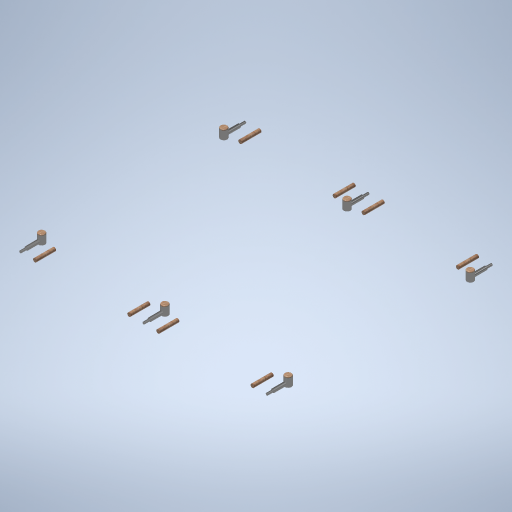
# Autodesk Inventor part: REC_01
Saved by Autodesk Inventor 2024.3 (Build 283343000, 343)
## iProperties
RuleStatus: InUse
Created: 2014-05-08
Part Number: REC_01
Material: Generic
Document SubType Name: Modeling
Designer: SauliusD
Density: 1 g/cm^3
Appearance: Default
Description: Pillar Board & 2 Nestled Boards from Sides Minifixes-01
AfterDocNew0: Fire Form
Author: SauliusD
Autodesk Inventor part; units mm, degrees
sketch "Sketch2" plane through (0, 0, 0) normal (0, 0, 1) x (1, 0, 0)
  line L0 (687.7589, -308.1253) -> (141.7589, -308.1253)
  line L1 (141.7589, -308.1253) -> (141.7589, 161.8747)
  line L2 (141.7589, 161.8747) -> (687.7589, 161.8747)
  line L3 (687.7589, 161.8747) -> (687.7589, -308.1253)
  point P0 (414.7589, 161.8747)
  point P1 (141.7589, -73.1253)
  constraints: 8 end point, 2 midpoint, 2 parallel, 1 horizontal, 1 perpendicular
ref_plane "Work Plane1" through (0, 0, -12.5) normal (0, 0, 1) x (1, 0, 0)
sketch "Sketch3" plane through (0, 0, -12.5) normal (0, 0, 1) x (1, 0, 0)
  line L0 (687.7589, 161.8747) -> (687.7589, -308.1253) construction
  line L1 (141.7589, 161.8747) -> (687.7589, 161.8747) construction
  line L2 (141.7589, -308.1253) -> (141.7589, 161.8747) construction
  line L3 (142.7589, 161.8747) -> (146.7589, 161.8747)
  line L4 (146.7589, 161.8747) -> (146.7589, 127.8747)
  line L5 (146.7589, 127.8747) -> (142.7589, 127.8747)
  line L6 (142.7589, 127.8747) -> (142.7589, 161.8747)
  line L7 (142.7589, 161.8747) -> (145.2589, 161.8747)
  line L8 (145.2589, 161.8747) -> (145.2589, 174.8747)
  line L9 (145.2589, 174.8747) -> (142.7589, 174.8747)
  line L10 (142.7589, 174.8747) -> (142.7589, 161.8747)
  line L11 (414.7589, 161.8747) -> (414.7589, 132.7708) construction
  line L12 (686.7589, 127.8747) -> (686.7589, 161.8747)
  point P0 (0, 0)
  dimension "d5" = 8
  dimension "d7" = 5
  dimension "d8" = 13
  dimension "Dist_Between_Planes" = 546
  dimension "Distance_between_Axis" = 544
  constraints: 20 end point, 5 parallel, 2 horizontal, 2 perpendicular, 2 symmetric about line, 1 collinear, 1 midpoint, 1 vertical alignment
  measures "d5" diameter of L4 L6
  measures "d7" diameter of L8 L10
  measures "d8" distance of L7.end L8.end
  measures "Dist_Between_Planes" distance of L1.start L0.start
  measures "Distance_between_Axis" distance between parallel lines of L6 L12
revolve "Minifix Revolve" add sketch "Sketch3" angle 360 about axis through (142.7589, 174.8747, -12.5) along (0, -1, 0)
sketch "Sketch4" plane through (0, 0, -12.5) normal (0, 0, 1) x (1, 0, 0)
  line L0 (138.7589, 127.8747) -> (146.7589, 127.8747) construction
  circle A0 centre (142.7589, 127.8747) radius 7.5
  point P0 (0, 0)
  dimension "d10" = 15
  constraints: 1 centre point, 1 midpoint
  measures "d10" diameter of A0
extrude "Minifix Extrude" add sketch "Sketch4" along normal up to surface (12.5 mm away)
extrude "Minifix extrude 2" add sketch "Sketch4" against normal blind 6
ref_plane "Work Plane2" through (414.7589, 161.8747, 0) normal (1, 0, 0) x (0, 1, 0)
ref_plane "Work Plane3" through (141.7589, -73.1253, 0) normal (0, 1, 0) x (-1, 0, 0)
sketch "Sketch5" plane through (0, 0, -12.5) normal (0, 0, 1) x (1, 0, 0)
  line L0 (142.7589, 271.4747) -> (142.7589, -404.7253) construction
  line L1 (174.7589, 174.8747) -> (174.7589, 131.8747)
  line L2 (174.7589, 174.8747) -> (178.7589, 174.8747)
  line L3 (178.7589, 174.8747) -> (178.7589, 131.8747)
  line L4 (178.7589, 131.8747) -> (174.7589, 131.8747)
  line L5 (140.2589, 174.8747) -> (145.2589, 174.8747) construction
  line L6 (138.7589, 161.8747) -> (146.7589, 161.8747) construction
  point P0 (0, 0)
  dimension "Dowel_D" = 8
  dimension "Dowel_Drill_Depth" = 30
  dimension "d17" = 32
  constraints: 8 end point, 2 parallel, 2 perpendicular, 1 collinear
  measures "Dowel_D" diameter of L3 L1
  measures "Dowel_Drill_Depth" distance between parallel lines of L4 L6
  measures "d17" distance from line of L1.start L0
revolve "Dowel Revolve" add sketch "Sketch5" angle 360 about axis through (174.7589, 174.8747, -12.5) along (0, -1, 0) separate body
mirror "Mirror1" about plane through (414.7589, 161.8747, 0) normal (1, 0, 0) of "Minifix Extrude", "Minifix Revolve", "Dowel Revolve", "Minifix extrude 2" bodies 1
sketch "Sketch6" plane through (0, 0, -12.5) normal (0, 0, 1) x (1, 0, 0)
  point P0 (0, 0)
sketch "Sketch7" plane through (0, 0, -12.5) normal (0, 0, 1) x (1, 0, 0)
  line L0 (414.7589, 271.4747) -> (414.7589, -404.7253) construction
  line L1 (417.2589, 161.8747) -> (414.7589, 161.8747)
  line L2 (414.7589, 161.8747) -> (414.7589, 174.8747)
  line L3 (414.7589, 174.8747) -> (417.2589, 174.8747)
  line L4 (417.2589, 174.8747) -> (417.2589, 161.8747)
  line L5 (414.7589, 161.8747) -> (418.7589, 161.8747)
  line L6 (418.7589, 161.8747) -> (418.7589, 127.8747)
  line L7 (418.7589, 127.8747) -> (414.7589, 127.8747)
  line L8 (414.7589, 127.8747) -> (414.7589, 161.8747)
  line L9 (140.2589, 174.8747) -> (145.2589, 174.8747) construction
  line L10 (138.7589, 161.8747) -> (146.7589, 161.8747) construction
  point P0 (0, 0)
  point P1 (414.7589, -404.7253)
  dimension "d19" = 34
  dimension "d20" = 5
  dimension "d21" = 8
  constraints: 16 end point, 4 parallel, 2 collinear, 2 horizontal, 2 perpendicular, 1 vertical, 1 other
  measures "d19" distance of L5.end L6.end
  measures "d20" diameter of L4 L2
  measures "d21" diameter of L6 L2
revolve "Center minixix Revolution" add sketch "Sketch7" angle 360 about axis through (414.7589, 161.8747, -12.5) along (0, 1, 0) separate body
sketch "Sketch8" plane through (0, 0, -12.5) normal (0, 0, 1) x (1, 0, 0)
  circle A0 centre (414.7589, 127.8747) radius 7.5
  line L0 (418.7589, 127.8747) -> (414.7589, 127.8747) construction
  point P0 (0, 0)
  dimension "d23" = 15
  constraints: 1 centre point, 1 coincident
  measures "d23" diameter of A0
extrude "Center minixix Extrusion 1" add sketch "Sketch8" along normal up to surface (12.5 mm away) bodies 3
extrude "Center minixix Extrusion 2" add sketch "Sketch8" against normal up to surface (6 mm away) bodies 3
ref_plane "Work Plane4" through (687.7589, 161.8747, 0) normal (0, 1, 0) x (-1, 0, 0)
mirror "Mirror2" about plane through (141.7589, -73.1253, 0) normal (0, 1, 0) of "Minifix Extrude", "Minifix Revolve", "Dowel Revolve", "Minifix extrude 2", "Mirror1" bodies 1
mirror "Mirror Center" about plane through (141.7589, -73.1253, 0) normal (0, 1, 0) of "Center minixix Revolution", "Center minixix Extrusion 1", "Center minixix Extrusion 2" bodies 3
sketch "Sketch9" plane through (142.7589, 127.8747, 0) normal (0, 0, 1) x (1, 0, 0)
  circle A0 centre (0, 0) radius 7.5 projected
  point P0 (-142.7589, -127.8747)
extrude "Side Cover Cap Extrusion" add sketch "Sketch9" along normal blind 2 separate body
fillet "Side Cover Cap Fillet" radius 1.6 1 edges at (135.2589, 127.8747, 2)
mirror "Mirror3" about plane through (414.7589, 161.8747, 0) normal (1, 0, 0) of "Side Cover Cap Extrusion", "Side Cover Cap Fillet" bodies 4
mirror "Mirror4" about plane through (141.7589, -73.1253, 0) normal (0, 1, 0) of "Side Cover Cap Extrusion", "Side Cover Cap Fillet", "Mirror3" bodies 4
sketch "Sketch10" plane through (0, 0, 0) normal (0, 0, 1) x (1, 0, 0)
  circle A0 centre (414.7589, 127.8747) radius 7.5
  line L0 (141.7589, 161.8747) -> (687.7589, 161.8747) projected
  point P0 (18.2411, -127.8747)
  point P1 (414.7589, 161.8747)
  dimension "d42" = 34
  constraints: 1 centre point, 1 midpoint, 1 vertical alignment
  measures "d42" distance from line of L0 A0.centre
extrude "Center Cover Cap Extrusion" add sketch "Sketch10" along normal blind 2 separate body
fillet "Center Cover Cap Fillet" radius 1.6 1 edges at (407.2589, 127.8747, 2)
mirror "Mirror5" about plane through (141.7589, -73.1253, 0) normal (0, 1, 0) of "Center Cover Cap Extrusion", "Center Cover Cap Fillet" bodies 5
sketch "Sketch11" plane through (0, 0, -12.5) normal (0, 0, 1) x (1, 0, 0)
  line L0 (414.7589, 258.4747) -> (414.7589, -417.7253) construction
  line L1 (378.7589, -321.1253) -> (382.7589, -321.1253)
  line L2 (382.7589, -321.1253) -> (382.7589, -278.1253)
  line L3 (382.7589, -278.1253) -> (378.7589, -278.1253)
  line L4 (378.7589, -278.1253) -> (378.7589, -321.1253)
  line L5 (658.7589, -321.1253) -> (650.7589, -321.1253) construction
  line L6 (658.7589, -278.1253) -> (650.7589, -278.1253) construction
  point P0 (0, 0)
  dimension "d43" = 8
  dimension "d44" = 32
  constraints: 8 end point, 2 collinear, 2 parallel, 1 horizontal, 1 perpendicular
  measures "d43" diameter of L4 L2
  measures "d44" distance from line of L1.end L0
revolve "Center Dowel Revolve" add sketch "Sketch11" angle 360 about axis through (382.7589, -321.1253, -12.5) along (0, 1, 0) bodies 1
mirror "Mirror7" about plane through (414.7589, 161.8747, 0) normal (1, 0, 0) of "Center Dowel Revolve" bodies 1
mirror "Mirror8" about plane through (141.7589, -73.1253, 0) normal (0, 1, 0) of "Center Dowel Revolve", "Mirror7" bodies 1
equation "\"d23\" = d10"
equation "\"d38\" = d35"
equation "\"d20\" = d7"
equation "\"d21\" = d5"
equation "\"d43\" = Dowel_D"
equation "\"d44\" = Step"
equation "\"Step\" = 32"
equation "\"d35\" = 1.6"
